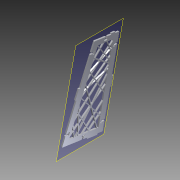
# Autodesk Inventor part: Panel_side
Saved by Autodesk Inventor 2013 (Build 170138000, 138)
## iProperties
Created: 2013-02-02
Part Number: Panel_side
Material: Aluminum 6061
Document SubType Name: Modeling
Designer: xylzlyx
Density: 1 g/cm^3
ScrewLen: 0.475 in
ScrewHoleD: 0.150 in
NutFlatsGap: 0.323 in
NutHeightGap: 0.119 in
SlotFilletRad: 0.020 in
ScrewHoleDist: 1.000 in
MetalThickness: 0.125 in
SlotWidth: 0.145 in
TabLength: 1.000 in
SlotLength: 1.020 in
SmallSlotLength: 0.395 in
SmallTabLength: 0.375 in
EdgeThickness: 0.500 in
Author: xylzlyx
Autodesk Inventor part; units mm, degrees
ref_plane "YZ Plane" through (0, 0, 0) normal (1, 0, 0) x (0, 1, 0)
ref_plane "XZ Plane" through (0, 0, 0) normal (0, 1, 0) x (-1, 0, 0)
ref_plane "XY Plane" through (0, 0, 0) normal (0, 0, 1) x (1, 0, 0)
ref_plane "Work Plane1" through (-221.4413, -90.9255, -118.1004) normal (-0.9848078, 0.1736482, 0) x (-0.1736482, -0.9848078, 0)
sketch "Sketch1" plane through (-221.4413, -90.9255, -118.1004) normal (-0.9848078, 0.1736482, 0) x (-0.1736482, -0.9848078, 0)
  line L0 (0, 0) -> (-0.5513, 3.1268) construction
  line L1 (-0.5513, 3.1268) -> (245.7896, 46.5633) construction
  line L2 (245.7896, 46.5633) -> (246.341, 43.4366) construction
  line L3 (246.341, 43.4366) -> (0, 0) construction
  line L4 (254.4978, -57.6752) -> (251.371, -58.2265) construction
  line L5 (251.371, -58.2265) -> (233.8339, 41.2312) construction
  line L6 (233.8339, 41.2312) -> (236.9607, 41.7826) construction
  line L7 (236.9607, 41.7826) -> (254.4978, -57.6752) construction
  line L8 (12.5071, 2.2053) -> (23.1628, -58.2265) construction
  line L9 (23.1628, -58.2265) -> (20.0361, -58.7779) construction
  line L10 (20.0361, -58.7779) -> (9.3803, 1.654) construction
  line L11 (9.3803, 1.654) -> (12.5071, 2.2053) construction
  line L12 (264.2669, -61.4015) -> (10.2669, -61.4015) construction
  line L13 (10.2669, -61.4015) -> (10.2669, -58.2265) construction
  line L14 (10.2669, -58.2265) -> (264.2669, -58.2265) construction
  line L15 (264.2669, -58.2265) -> (264.2669, -61.4015) construction
  line L16 (233.8339, 41.2312) -> (251.371, -58.2265)
  line L17 (251.371, -58.2265) -> (23.1628, -58.2265)
  line L18 (23.1628, -58.2265) -> (12.5071, 2.2053)
  line L19 (12.5071, 2.2053) -> (233.8339, 41.2312)
  point P0 (-127.997, 118.1004)
  constraints: 40 end point, 4 collinear, 2 horizontal, 2 vertical, 28 other
extrude "SidePanel" add sketch "Sketch1" against normal blind 3.175
fillet "CornerFillet" radius 1 4 edges at (-263.5281, -338.7532, -176.327) (-260.4828, -321.4826, -76.8692) (-223.9001, -114.0121, -176.327) (-222.0498, -103.5182, -115.8951)
sketch "ScrewSketch" plane through (-221.4413, -90.9255, -118.1004) normal (-0.9848078, 0.1736482, 0) x (0, 0, 1)
  line L0 (-57.0529, -251.164) -> (40.2464, -234.0076) projected
  line L1 (41.0576, -232.8491) -> (2.379, -13.4919) projected
  line L2 (-61.4015, -11.2669) -> (-61.4015, -263.2669) projected
  line L3 (-58.2265, -250.1792) -> (-58.2265, -24.0019) projected
  line L4 (-61.4015, -226.6779) -> (-49.3365, -226.6779)
  line L5 (-61.4015, -222.8806) -> (-49.3365, -222.8806)
  line L6 (-61.4015, -222.8806) -> (-61.4015, -226.6779)
  line L7 (-49.3365, -226.6779) -> (-49.3365, -222.8806)
  line L8 (-61.4015, -47.5033) -> (-49.3365, -47.5033)
  line L9 (-49.3365, -47.5033) -> (-49.3365, -51.3006)
  line L10 (-49.3365, -51.3006) -> (-61.4015, -51.3006)
  line L11 (-61.4015, -51.3006) -> (-61.4015, -47.5033)
  line L12 (3.3004, -0.4335) -> (46.3897, -244.8048) projected
  line L13 (-2.295, -38.1799) -> (9.5867, -36.0848)
  line L14 (-2.295, -38.1799) -> (-1.6356, -41.9195)
  line L15 (-1.6356, -41.9195) -> (10.2461, -39.8245)
  line L16 (10.2461, -39.8245) -> (9.5867, -36.0848)
  line L17 (28.2217, -211.2485) -> (40.1034, -209.1535)
  line L18 (28.2217, -211.2485) -> (27.5623, -207.5089)
  line L19 (27.5623, -207.5089) -> (39.444, -205.4138)
  line L20 (39.444, -205.4138) -> (40.1034, -209.1535)
  line L21 (40.7978, -237.1343) -> (-56.6904, -254.3241) projected
  line L22 (0.6692, -9.5539) -> (-57.2417, -19.7652) projected
  line L23 (-49.3365, -228.875) -> (-49.3365, -220.6835)
  line L24 (-49.3365, -220.6835) -> (-52.3687, -220.6835)
  line L25 (-49.3365, -228.875) -> (-52.3687, -228.875)
  line L26 (-52.3687, -228.875) -> (-52.3687, -220.6835)
  line L27 (-49.3365, -45.3062) -> (-49.3365, -53.4977)
  line L28 (-49.3365, -53.4977) -> (-52.3687, -53.4977)
  line L29 (-52.3687, -53.4977) -> (-52.3687, -45.3062)
  line L30 (-52.3687, -45.3062) -> (-49.3365, -45.3062)
  line L31 (-1.2541, -44.0832) -> (-2.6765, -36.0162)
  line L32 (-1.2541, -44.0832) -> (1.732, -43.5567)
  line L33 (1.732, -43.5567) -> (0.3095, -35.4897)
  line L34 (0.3095, -35.4897) -> (-2.6765, -36.0162)
  line L35 (28.6032, -213.4122) -> (27.1808, -205.3452)
  line L36 (27.1808, -205.3452) -> (30.1668, -204.8187)
  line L37 (30.1668, -204.8187) -> (31.5893, -212.8857)
  line L38 (31.5893, -212.8857) -> (28.6032, -213.4122)
  line L39 (-6.0765, -245.3995) -> (-8.1716, -233.5178)
  line L40 (-11.9112, -234.1772) -> (-9.8161, -246.0589)
  line L41 (-8.1716, -233.5178) -> (-11.9112, -234.1772)
  line L42 (-6.0765, -245.3995) -> (-9.8161, -246.0589)
  line L43 (-14.0749, -234.5587) -> (-6.0079, -233.1363)
  line L44 (-13.5484, -237.5448) -> (-14.0749, -234.5587)
  line L45 (-13.5484, -237.5448) -> (-5.4813, -236.1223)
  line L46 (-5.4813, -236.1223) -> (-6.0079, -233.1363)
  line L47 (-26.4165, -14.3299) -> (-24.3214, -26.2116)
  line L48 (-24.3214, -26.2116) -> (-28.061, -26.871)
  line L49 (-28.061, -26.871) -> (-30.1561, -14.9893)
  line L50 (-30.1561, -14.9893) -> (-26.4165, -14.3299)
  line L51 (-30.2247, -27.2525) -> (-22.1577, -25.8301)
  line L52 (-22.1577, -25.8301) -> (-22.6842, -22.844)
  line L53 (-22.6842, -22.844) -> (-30.7513, -24.2664)
  line L54 (-30.7513, -24.2664) -> (-30.2247, -27.2525)
  line L55 (-61.4015, -224.7792) -> (-49.3365, -224.7792) construction
  line L56 (-61.4015, -49.4019) -> (-49.3365, -49.4019) construction
  line L57 (9.9164, -37.9547) -> (-1.9653, -40.0497) construction
  line L58 (39.7737, -207.2836) -> (27.892, -209.3787) construction
  point P0 (-7.9463, -245.7292)
  point P1 (-10.0414, -233.8475)
  point P2 (-28.2863, -14.6596)
  point P3 (-26.1912, -26.5413)
  dimension "d7" = 12.065
  dimension "d8" = 3.7973
  dimension "d10" = 12.065
  dimension "d11" = 3.7973
  dimension "d14" = 12.065
  dimension "d17" = 3.7973
  dimension "d18" = 12.065
  dimension "d20" = 3.7973
  dimension "d21" = 8.1915
  dimension "d22" = 3.0321
  dimension "d23" = 8.1915
  dimension "d24" = 3.0321
  dimension "d25" = 8.1915
  dimension "d26" = 3.0321
  dimension "d27" = 8.1915
  dimension "d28" = 3.0321
  dimension "d29" = 12.065
  dimension "d30" = 3.7973
  dimension "d31" = 8.1915
  dimension "d32" = 3.0321
  dimension "d33" = 3.7973
  dimension "d34" = 12.065
  dimension "d35" = 8.1915
  dimension "d36" = 3.0321
  dimension "d40" = 25.4
  dimension "d41" = 25.4
  dimension "d42" = 25.4
  dimension "d43" = 25.4
  constraints: 104 end point, 39 parallel, 16 midpoint, 9 collinear, 6 perpendicular, 6 point on line
  measures "d7" distance of L4.start L4.end
  measures "d8" distance between parallel lines of L4 L5
  measures "d10" distance of L8.start L8.end
  measures "d11" distance of L10.end L8.start
  measures "d14" distance of L13.start L13.end
  measures "d17" distance between parallel lines of L13 L15
  measures "d18" distance of L17.start L17.end
  measures "d20" distance of L19.end L17.end
  measures "d21" distance of L23.start L23.end
  measures "d22" distance of L23.end L24.end
  measures "d23" distance of L27.start L27.end
  measures "d24" distance of L27.end L28.end
  measures "d25" distance of L31.start L31.end
  measures "d26" distance of L31.start L32.end
  measures "d27" distance of L35.start L35.end
  measures "d28" distance of L35.end L36.end
  measures "d29" distance of L39.start L39.end
  measures "d30" distance of L39.end L40.start
  measures "d31" distance of L43.start L43.end
  measures "d32" distance of L44.start L43.start
  measures "d33" distance of L49.end L47.start
  measures "d34" distance of L48.end L49.end
  measures "d35" distance of L51.start L51.end
  measures "d36" distance of L51.end L52.end
  measures "d40" vertical distance of L55.start L3.start
  measures "d41" vertical distance of L3.end L56.start
  measures "d42" distance from line of L1.end L57
  measures "d43" distance from line of L1.start L58
extrude "ScrewSlots" cut sketch "ScrewSketch" against normal blind 25.4 contours L40 L45 L39 L0 | L0 L39 L21 L40 | L45 L44 L43 L40 | L40 L41 L39 L45 | L39 L43 L46 L45 | L17 L37 L19 L1 | L1 L19 L12 L17 | L37 L38 L35 L17 | L17 L18 L19 L37 | L15 L33 L13 L1 | L1 L13 L12 L15 | L19 L35 L36 L37 | L33 L32 L31 L15 | L15 L14 L13 L33 | L13 L31 L34 L33 | L8 L3 L10 L2 | L8 L29 L10 L3 | L5 L3 L4 L2 | L29 L30 L27 L8 | L8 L9 L10 L29 | L5 L26 L4 L3 | L10 L27 L28 L29 | L26 L24 L23 L5 | L5 L7 L4 L26 | L4 L23 L25 L26 | L47 L53 L49 L22 | L53 L52 L51 L47 | L47 L48 L49 L53 | L49 L51 L54 L53
fillet "SlotFillets" radius 0.5 48 edges at (-261.9482, -329.7932, -124.7283) (-260.9464, -324.112, -125.7455) (-262.0627, -330.4426, -128.4679) (-261.0609, -324.7613, -129.4851) (-261.1272, -325.1371, -131.6488) (-260.6087, -322.1964, -132.1754) (-260.3617, -320.7956, -124.1083) (-260.8802, -323.7362, -123.5818) (-256.4695, -298.7218, -86.8927) (-256.8452, -300.8526, -86.5112) (-256.9366, -301.3712, -89.4972) (-255.5358, -293.4267, -90.9197) (-255.4443, -292.9081, -87.9336) (-255.8201, -295.039, -87.5521) (-256.2928, -297.72, -81.1238) (-255.6434, -294.0372, -81.7832) (-259.6217, -316.599, -167.437) (-259.6217, -316.599, -170.4691) (-259.2402, -314.4353, -170.4691) (-259.2402, -314.4353, -176.327) (-258.5808, -310.6957, -176.327) (-258.5808, -310.6957, -170.4691) (-258.1992, -308.5319, -170.4691) (-258.1992, -308.5319, -167.437) (-229.1677, -143.8861, -167.437) (-229.1677, -143.8861, -170.4691) (-228.7862, -141.7223, -170.4691) (-228.7862, -141.7223, -176.327) (-228.1268, -137.9827, -176.327) (-228.1268, -137.9827, -170.4691) (-227.7453, -135.819, -170.4691) (-227.7453, -135.819, -167.437) (-224.6103, -118.0396, -148.3252) (-224.3633, -116.6388, -140.2581) (-223.8448, -113.6981, -140.7846) (-223.911, -114.0738, -142.9484) (-224.0255, -114.7232, -146.688) (-224.0918, -115.0989, -148.8517) (-223.0238, -109.0419, -147.7052) (-222.9093, -108.3926, -143.9656) (-226.1321, -126.6701, -120.777) (-227.4415, -134.0961, -116.3685) (-227.5329, -134.6146, -119.3545) (-226.0407, -126.1516, -117.7909) (-226.2398, -127.2807, -111.6405) (-226.8891, -130.9635, -110.9811) (-226.4164, -128.2825, -117.4094) (-227.0658, -131.9653, -116.75)
sketch "TopTabSketch" plane through (-260.0573, -309.9276, -176.327) normal (0, 0, -1) x (-0.9848078, 0.1736482, 0)
  line L0 (0, 72.59) -> (-3.175, 72.59)
  line L1 (-3.175, 72.59) -> (-3.175, 97.99)
  line L2 (-3.175, 97.99) -> (0, 97.99)
  line L3 (0, 97.99) -> (0, 72.59)
  line L4 (0.254, 72.836) -> (0.254, 97.744) projected
  line L5 (-2.929, 72.336) -> (-0.246, 72.336) projected
  point P0 (-3.175, -27.7987)
  point P1 (0, 85.29)
  point P2 (0.254, 85.29)
  point P3 (-1.5875, 72.59)
  point P4 (-1.5875, 72.336)
  dimension "d44" = 25.4
  constraints: 8 end point, 4 midpoint, 2 parallel, 2 vertical alignment, 1 horizontal, 1 horizontal alignment, 1 perpendicular
  measures "d44" distance of L0.end L1.end
extrude "TopTab" add sketch "TopTabSketch" along normal blind 3.175
fillet "TopTabFillet" radius 0.5 4 edges at (-245.8888, -238.7161, -179.502) (-245.8888, -238.7161, -176.327) (-241.4782, -213.7019, -179.502) (-241.4782, -213.7019, -176.327)
sketch "BottomTabSketch" plane through (-257.1213, -293.2766, -81.87) normal (0.0301537, 0.1710101, 0.9848078) x (0.9848078, -0.1736482, 0)
  line L0 (3.175, 96.2719) -> (0, 96.2719)
  line L1 (0, 96.2719) -> (0, 70.8719)
  line L2 (0, 70.8719) -> (3.175, 70.8719)
  line L3 (3.175, 70.8719) -> (3.175, 96.2719)
  line L4 (2.929, 96.5259) -> (0.246, 96.5259) projected
  line L5 (-0.254, 96.0259) -> (-0.254, 71.1179) projected
  point P0 (3.175, 167.1439)
  point P1 (202.2881, 314.187)
  point P2 (0, 83.5719)
  point P3 (-0.254, 83.5719)
  point P4 (1.5875, 96.2719)
  point P5 (1.5875, 96.5259)
  dimension "d50" = 25.4
  constraints: 8 end point, 4 midpoint, 2 parallel, 2 vertical alignment, 1 horizontal, 1 horizontal alignment, 1 perpendicular
  measures "d50" distance of L2.end L0.start
extrude "BottomTab" add sketch "BottomTabSketch" along normal blind 3.175
fillet "BottomTabFillet" radius 0.5 4 edges at (-239.0945, -200.1833, -98.5875) (-238.9987, -199.6404, -95.4607) (-243.3424, -224.2745, -91.0501) (-243.4381, -224.8174, -94.1768)
sketch "BackTabSketch" plane through (-265.0555, -338.2738, -175.1533) normal (-0.1710101, -0.9698463, 0.1736482) x (0.9848078, -0.1736482, 0)
  line L0 (0, 11.3563) -> (3.175, 11.3563)
  line L1 (3.175, 11.3563) -> (3.175, 36.7563)
  line L2 (3.175, 36.7563) -> (0, 36.7563)
  line L3 (0, 36.7563) -> (0, 11.3563)
  line L4 (2.929, 37.0103) -> (0.246, 37.0103) projected
  line L5 (-0.254, 36.5103) -> (-0.254, 11.6023) projected
  point P0 (0, 0)
  point P1 (202.2881, 238.333)
  point P2 (-0.254, 24.0563)
  point P3 (0, 24.0563)
  point P4 (1.5875, 36.7563)
  point P5 (1.5875, 37.0103)
  dimension "d56" = 25.4
  constraints: 8 end point, 4 midpoint, 2 parallel, 2 vertical alignment, 1 horizontal, 1 horizontal alignment, 1 perpendicular
  measures "d56" distance of L0.end L1.end
extrude "BackTab" add sketch "BackTabSketch" along normal blind 3.175
fillet "BackTabFillet" radius 0.5 4 edges at (-262.3838, -332.2637, -138.9555) (-262.9268, -335.343, -138.4042) (-263.6927, -339.6867, -163.4183) (-263.1497, -336.6074, -163.9696)
sketch "FrontTabSketch" plane through (-225.4382, -113.5929, -175.5006) normal (0.1710101, 0.9698463, -0.1736482) x (0.9848078, -0.1736482, 0)
  line L0 (3.175, -10.1593) -> (0, -10.1593)
  line L1 (0, -10.1593) -> (0, -19.6843)
  line L2 (0, -19.6843) -> (3.175, -19.6843)
  line L3 (3.175, -19.6843) -> (3.175, -10.1593)
  line L4 (2.929, -9.9053) -> (0.246, -9.9053) projected
  line L5 (-0.254, -10.4053) -> (-0.254, -19.4383) projected
  point P0 (3.175, 0)
  point P1 (202.2881, -199.0577)
  point P2 (0, -14.9218)
  point P3 (-0.254, -14.9218)
  point P4 (1.5875, -10.1593)
  point P5 (1.5875, -9.9053)
  dimension "d61" = 9.525
  constraints: 8 end point, 4 midpoint, 2 parallel, 2 vertical alignment, 1 horizontal, 1 horizontal alignment, 1 perpendicular
  measures "d61" distance of L2.end L0.start
extrude "FrontTab" add sketch "FrontTabSketch" along normal blind 3.175
fillet "FrontTabFillet" radius 0.5 4 edges at (-223.5685, -112.1312, -165.4957) (-223.0255, -109.052, -166.047) (-222.7383, -107.4231, -156.6667) (-223.2813, -110.5023, -156.1154)
sketch "Sketch7" plane through (-221.4413, -90.9255, -118.1004) normal (-0.9848078, 0.1736482, 0) x (0, 0, 1)
  line L0 (-47.8876, -21.3398) -> (-57.4002, -23.0171) projected
  line L1 (-58.2265, -24.0019) -> (-58.2265, -47.0033) projected
  line L2 (-58.2265, -227.1779) -> (-58.2265, -250.1792) projected
  line L3 (-57.0529, -251.164) -> (-46.3616, -249.2789) projected
  line L4 (-6.1355, -242.1859) -> (40.2464, -234.0076) projected
  line L5 (41.0576, -232.8491) -> (37.0634, -210.1972) projected
  line L6 (6.3731, -36.1438) -> (2.379, -13.4919) projected
  line L7 (1.2205, -12.6807) -> (-25.3727, -17.3698) projected
  line L8 (-45.5265, -236.2357) -> (26.5188, -223.5322)
  line L9 (26.5188, -223.5322) -> (-8.0964, -27.2194)
  line L10 (-8.0964, -27.2194) -> (-45.5265, -33.8194)
  line L11 (-45.5265, -33.8194) -> (-45.5265, -236.2357)
  point P0 (118.1004, 127.997)
  dimension "d66" = 12.7
  dimension "d67" = 12.7
  dimension "d68" = 12.7
  dimension "d69" = 12.7
  dimension "d70" = 12.7
  dimension "d71" = 12.7
  dimension "d72" = 12.7
  dimension "d73" = 12.7
  constraints: 8 end point
  measures "d66" distance from line of L8.start L2
  measures "d67" distance from line of L3 L8.start
  measures "d68" distance from line of L4 L8.end
  measures "d69" distance from line of L5 L8.end
  measures "d70" distance from line of L6 L9.end
  measures "d71" distance from line of L7 L9.end
  measures "d72" distance from line of L1 L10.end
  measures "d73" distance from line of L0 L10.end
extrude "InsideGap" cut sketch "Sketch7" against normal blind 3.175
fillet "InsideGapFillet" radius 0.5 4 edges at (-260.8999, -323.8479, -163.627) (-258.6939, -311.3373, -91.5816) (-224.6046, -118.0071, -126.1968) (-225.7506, -124.5067, -163.627)
sketch "Sketch8" plane through (-221.4413, -90.9255, -118.1004) normal (-0.9848078, 0.1736482, 0) x (0, 0, 1)
  line L0 (-8.0096, -27.7119) -> (26.432, -223.0398) projected
  line L1 (26.0264, -223.619) -> (-44.9397, -236.1322) projected
  line L2 (-45.5265, -235.6398) -> (-45.5265, -34.2389) projected
  line L3 (-45.1134, -33.7465) -> (-8.5888, -27.3063) projected
  line L4 (-21.4515, -231.9906) -> (-45.5265, -203.2991)
  line L5 (-7.0433, -229.4501) -> (-45.5265, -177.5946)
  line L6 (8.5655, -226.6978) -> (-45.5265, -118.5843)
  line L7 (25.4837, -217.6617) -> (-45.5265, -140.249)
  line L8 (19.6131, -184.3679) -> (-45.5265, -96.4651)
  line L9 (11.202, -136.666) -> (-45.5265, -74.8227)
  line L10 (5.4681, -104.1477) -> (-45.5265, -41.1745)
  line L11 (-1.0729, -67.0517) -> (-24.1897, -30.0571)
  line L12 (9.3495, -126.1601) -> (-45.5265, -102.8666)
  line L13 (2.6144, -87.9635) -> (-45.5265, -56.7004)
  line L14 (-19.1408, -231.5832) -> (-45.5265, -200.1378)
  line L15 (-4.8057, -229.0555) -> (-45.5265, -174.1849)
  line L16 (10.6534, -226.3297) -> (-45.5265, -114.043)
  line L17 (24.8275, -213.9404) -> (-45.5265, -137.243)
  line L18 (18.8234, -179.8894) -> (-45.5265, -93.0522)
  line L19 (10.5458, -132.9447) -> (-45.5265, -71.8167)
  line L20 (8.9288, -123.774) -> (-45.5265, -100.6591)
  line L21 (2.132, -85.2273) -> (-45.5265, -54.2775)
  line L22 (-2.0148, -61.7098) -> (-22.0314, -29.6766)
  line L23 (4.7403, -100.02) -> (-45.5265, -37.9456)
  line L24 (-19.1408, -231.5832) -> (-21.4515, -231.9906)
  line L25 (-45.5265, -200.1378) -> (-45.5265, -203.2991)
  line L26 (-45.5265, -174.1849) -> (-45.5265, -177.5946)
  line L27 (-7.0433, -229.4501) -> (-4.8057, -229.0555)
  line L28 (10.6534, -226.3297) -> (8.5655, -226.6978)
  line L29 (-45.5265, -137.243) -> (-45.5265, -140.249)
  line L30 (25.4837, -217.6617) -> (24.8275, -213.9404)
  line L31 (18.8234, -179.8894) -> (19.6131, -184.3679)
  line L32 (-45.5265, -114.043) -> (-45.5265, -118.5843)
  line L33 (-45.5265, -100.6591) -> (-45.5265, -102.8666)
  line L34 (-45.5265, -96.4651) -> (-45.5265, -93.0522)
  line L35 (11.202, -136.666) -> (10.5458, -132.9447)
  line L36 (9.3495, -126.1601) -> (8.9288, -123.774)
  line L37 (-45.5265, -71.8167) -> (-45.5265, -74.8227)
  line L38 (-45.5265, -56.7004) -> (-45.5265, -54.2775)
  line L39 (5.4681, -104.1477) -> (4.7403, -100.02)
  line L40 (2.6144, -87.9635) -> (2.132, -85.2273)
  line L41 (-1.0729, -67.0517) -> (-2.0148, -61.7098)
  line L42 (-45.5265, -41.1745) -> (-45.5265, -37.9456)
  line L43 (-22.0314, -29.6766) -> (-24.1897, -30.0571)
  dimension "d77" = 60
  dimension "d78" = 23.8506
  dimension "d79" = 38.481
  dimension "d80" = 63.42
  dimension "d81" = 54.3306
  dimension "d82" = 73.42
  dimension "d83" = 5.461
  dimension "d84" = 147.47
  dimension "d85" = 39.2684
  dimension "d86" = 153.46
  dimension "d87" = 87.7062
  dimension "d88" = 147.47
  dimension "d89" = 123
  dimension "d90" = 98.3742
  dimension "d91" = 120.7262
  dimension "d92" = 151
  dimension "d93" = 137.16
  dimension "d94" = 133
  dimension "d95" = 158.3944
  dimension "d96" = 158
  dimension "d97" = 2.032
  dimension "d98" = 2.032
  dimension "d99" = 2.032
  dimension "d100" = 2.032
  dimension "d101" = 2.032
  dimension "d102" = 2.032
  dimension "d103" = 2.032
  dimension "d104" = 2.032
  dimension "d106" = 2.032
  dimension "d107" = 2.032
  constraints: 80 end point, 10 parallel, 8 point on line, 34 other
  measures "d77" angle of L1 L4
  measures "d78" distance of L1.end L4.start
  measures "d79" distance of L1.end L5.start
  measures "d80" angle of L1 L5
  measures "d81" distance of L1.end L6.start
  measures "d82" angle of L1 L6
  measures "d83" distance of point (26.432, -223.04) L7.start
  measures "d85" distance of point (26.432, -223.04) L8.start
  measures "d87" distance of L9.start point (26.432, -223.04)
  measures "d90" distance of point (26.432, -223.04) L12.start
  measures "d91" distance of point (26.432, -223.04) L10.start
  measures "d93" distance of point (26.432, -223.04) L13.start
  measures "d95" distance of point (26.432, -223.04) L11.start
  measures "d97" distance between parallel lines of L4 L14
  measures "d98" distance between parallel lines of L5 L15
  measures "d99" distance between parallel lines of L6 L16
  measures "d100" distance between parallel lines of L7 L17
  measures "d101" distance between parallel lines of L8 L18
  measures "d102" distance between parallel lines of L9 L19
  measures "d103" distance between parallel lines of L12 L20
  measures "d104" distance between parallel lines of L13 L21
  measures "d106" distance between parallel lines of L11 L22
  measures "d107" distance between parallel lines of L10 L23
extrude "Hash1" add sketch "Sketch8" against normal blind 3.175 contours L0 L11 L3 L22 | L0 L13 L23 L21 | L23 L13 L10 L21 | L21 L10 L2 L23 | L0 L10 L13 L23 | L10 L13 L2 L21 | L0 L12 L19 L20 | L20 L9 L2 L19 | L19 L12 L9 L20 | L0 L9 L12 L19 | L9 L12 L18 L20 | L20 L8 L2 L18 | L18 L12 L8 L20 | L0 L8 L12 L18 | L8 L12 L2 L20 | L0 L7 L16 L17 | L17 L6 L2 L16 | L16 L7 L6 L17 | L16 L1 L6 L7 | L6 L7 L2 L17 | L1 L5 L2 L15 | L1 L4 L2 L14
sketch "Sketch9" plane through (-221.4413, -90.9255, -118.1004) normal (-0.9848078, 0.1736482, 0) x (0, 0, 1)
  line L0 (8.5655, -226.6978) -> (-4.8057, -229.0555) projected
  line L1 (-45.5265, -174.1849) -> (-45.5265, -140.249) projected
  line L2 (19.6131, -184.3679) -> (24.8275, -213.9404) projected
  line L3 (5.4681, -104.1477) -> (8.9288, -123.774) projected
  line L4 (-45.5265, -71.8167) -> (-45.5265, -56.7004) projected
  line L5 (-45.1134, -33.7465) -> (-24.1897, -30.0571) projected
  line L6 (-1.0729, -67.0517) -> (2.132, -85.2273) projected
  line L7 (-45.5265, -54.2775) -> (-45.5265, -41.1745) projected
  line L8 (-8.0096, -27.7119) -> (-2.0148, -61.7098) projected
  line L9 (26.0264, -223.619) -> (10.6534, -226.3297) projected
  line L10 (-21.4515, -231.9906) -> (-44.9397, -236.1322) projected
  line L11 (-45.5265, -235.6398) -> (-45.5265, -203.2991) projected
  line L12 (-45.5265, -93.0522) -> (-45.5265, -74.8227) projected
  line L13 (11.202, -136.666) -> (18.8234, -179.8894) projected
  line L14 (2.6144, -87.9635) -> (4.7403, -100.02) projected
  line L15 (20.8437, -191.3469) -> (12.7242, -225.9645)
  line L16 (16.0184, -163.9814) -> (-24.5043, -232.5289)
  line L17 (13.8263, -151.5494) -> (2.8521, -227.7053)
  line L18 (5.9798, -107.0493) -> (-43.25, -235.8343)
  line L19 (11.202, -136.666) -> (-45.5265, -207.0961)
  line L20 (1.3397, -80.7345) -> (-45.5265, -154.527)
  line L21 (-3.4988, -53.294) -> (-45.5265, -88.0007)
  line L22 (-8.1696, -26.804) -> (-45.5265, -80.1552)
  line L23 (-32.2561, -31.4795) -> (-45.5265, -58.6879)
  line L24 (21.7394, -196.4266) -> (14.9014, -225.5806)
  line L25 (12.7242, -225.9645) -> (14.9014, -225.5806)
  line L26 (21.7394, -196.4266) -> (20.8437, -191.3469)
  line L27 (4.9586, -227.3338) -> (14.9561, -157.9564)
  line L28 (4.9586, -227.3338) -> (2.8521, -227.7053)
  line L29 (14.9561, -157.9564) -> (13.8263, -151.5494)
  line L30 (-21.8691, -232.0643) -> (16.5608, -167.0571)
  line L31 (-40.9173, -235.423) -> (6.6665, -110.9438)
  line L32 (-40.9173, -235.423) -> (-43.25, -235.8343)
  line L33 (6.6665, -110.9438) -> (5.9798, -107.0493)
  line L34 (-45.5265, -210.3355) -> (11.6706, -139.3236)
  line L35 (11.6706, -139.3236) -> (11.202, -136.666)
  line L36 (-45.5265, -207.0961) -> (-45.5265, -210.3355)
  line L37 (-45.5265, -158.3172) -> (1.8628, -83.701)
  line L38 (1.8628, -83.701) -> (1.3397, -80.7345)
  line L39 (-45.5265, -158.3172) -> (-45.5265, -154.527)
  line L40 (-45.5265, -90.636) -> (-3.0931, -55.5943)
  line L41 (-3.0931, -55.5943) -> (-3.4988, -53.294)
  line L42 (-45.5265, -90.636) -> (-45.5265, -88.0007)
  line L43 (-45.5265, -83.6979) -> (-7.6706, -29.6341)
  line L44 (-7.6706, -29.6341) -> (-8.1696, -26.804)
  line L45 (-45.5265, -80.1552) -> (-45.5265, -83.6979)
  line L46 (-45.5265, -63.3232) -> (-29.7826, -31.0433)
  line L47 (-29.7826, -31.0433) -> (-32.2561, -31.4795)
  line L48 (-45.5265, -58.6879) -> (-45.5265, -63.3232)
  line L49 (-21.8691, -232.0643) -> (-24.5043, -232.5289)
  point P0 (26.432, -223.0398)
  point P1 (118.1004, 127.997)
  dimension "d110" = 32.1818
  dimension "d111" = 23.2
  dimension "d112" = 59.9694
  dimension "d113" = 40.59
  dimension "d114" = 72.5932
  dimension "d115" = 18.2
  dimension "d116" = 87.7062
  dimension "d117" = 48.85
  dimension "d118" = 117.7798
  dimension "d119" = 30.92
  dimension "d120" = 144.5006
  dimension "d121" = 42.42
  dimension "d122" = 172.3644
  dimension "d123" = 60.45
  dimension "d124" = 199.263
  dimension "d125" = 45
  dimension "d126" = 13.0556
  dimension "d127" = 126
  dimension "d128" = 2.032
  dimension "d129" = 2.032
  dimension "d131" = 2.032
  dimension "d132" = 2.032
  dimension "d133" = 2.032
  dimension "d134" = 2.032
  dimension "d135" = 2.032
  dimension "d136" = 2.032
  dimension "d137" = 2.032
  constraints: 70 end point, 29 point on line, 9 parallel, 8 other
  measures "d110" distance of point (26.432, -223.04) L15.start
  measures "d111" angle of L2 L15
  measures "d112" distance of point (26.432, -223.04) L16.start
  measures "d114" distance of point (26.432, -223.04) L17.start
  measures "d116" distance of point (26.432, -223.04) L19.start
  measures "d118" distance of point (26.432, -223.04) L18.start
  measures "d119" angle of L3 L18
  measures "d120" distance of point (26.432, -223.04) L20.start
  measures "d121" angle of L14 L20
  measures "d122" distance of point (26.432, -223.04) L21.start
  measures "d123" angle of L6 L21
  measures "d124" distance of point (26.432, -223.04) L22.start
  measures "d125" angle of L8 L22
  measures "d126" distance of L23.start L5.start
  measures "d127" angle of L5 L23
  measures "d128" distance between parallel lines of L15 L24
  measures "d129" distance between parallel lines of L17 L27
  measures "d131" distance between parallel lines of L18 L31
  measures "d132" distance between parallel lines of L19 L34
  measures "d133" distance between parallel lines of L20 L37
  measures "d134" distance between parallel lines of L21 L40
  measures "d135" distance between parallel lines of L22 L43
  measures "d136" distance between parallel lines of L23 L46
  measures "d137" distance between parallel lines of L16 L30
extrude "Hash2" add sketch "Sketch9" against normal blind 3.175 contours L0 L17 L30 L27 | L30 L17 L16 L27 | L27 L16 L13 L30 | L30 L10 L16 L17 | L16 L17 L13 L27 | L10 L18 L34 L31 | L34 L31 L19 L13 | L34 L18 L19 L31 | L34 L11 L19 L18 | L19 L18 L3 L31 | L1 L20 L6 L37 | L2 L24 L9 L15 | L4 L23 L5 L46 | L8 L43 L12 L22 L44 | L8 L40 L12 L21
equation "\"d7\" = ScrewLen"
equation "\"d8\" = ScrewHoleD"
equation "\"d10\" = ScrewLen"
equation "\"d11\" = ScrewHoleD"
equation "\"d14\" = ScrewLen"
equation "\"d17\" = ScrewHoleD"
equation "\"d18\" = ScrewLen"
equation "\"d20\" = ScrewHoleD"
equation "\"d21\" = NutFlatsGap"
equation "\"d22\" = NutHeightGap"
equation "\"d23\" = NutFlatsGap"
equation "\"d24\" = NutHeightGap"
equation "\"d25\" = NutFlatsGap"
equation "\"d26\" = NutHeightGap"
equation "\"d27\" = NutFlatsGap"
equation "\"d28\" = NutHeightGap"
equation "\"d29\" = ScrewLen"
equation "\"d30\" = ScrewHoleD"
equation "\"d31\" = NutFlatsGap"
equation "\"d32\" = NutHeightGap"
equation "\"d33\" = ScrewHoleD"
equation "\"d34\" = ScrewLen"
equation "\"d35\" = NutFlatsGap"
equation "\"d36\" = NutHeightGap"
equation "\"ScrewLen\" = 12.065"
equation "\"ScrewHoleD\" = 3.7973"
equation "\"NutFlatsGap\" = 8.1915"
equation "\"NutHeightGap\" = 3.03212"
equation "\"SlotFilletRad\" = 0.5"
equation "\"ScrewHoleDist\" = 25.4"
equation "\"MetalThickness\" = 3.175"
equation "\"SlotWidth\" = 3.683"
equation "\"TabLength\" = 25.4"
equation "\"SlotLength\" = 25.908"
equation "\"SmallSlotLength\" = 10.033"
equation "\"SmallTabLength\" = 9.525"
equation "\"WasherHeight\" = 1.27"
equation "\"EdgeThickness\" = 12.7"
equation "\"GridThickness\" = 2.032"
body "Solid1"
